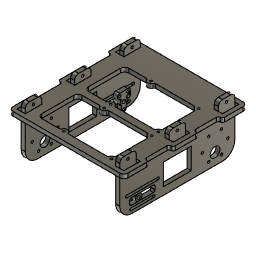
scocca v1.4 (Autodesk Fusion 360 design; units mm, degrees)
Autodesk Fusion 360 part; units mm, degrees
sketch "Schizzo1" plane through (0, 0, 0) normal (0, 0, 1) x (1, 0, 0)
  circle A0 centre (36.25, 84.4234) radius 1.5
  circle A1 centre (28.5, 71) radius 1.5
  circle A2 centre (36.25, 57.5766) radius 1.5
  circle A3 centre (59.5, 71) radius 1.5
  circle A4 centre (51.75, 57.5766) radius 1.5
  circle A5 centre (51.75, 84.4234) radius 1.5
  circle A6 centre (44, 64) radius 6
  line L0 (19.9998, 100) -> (19.9998, 65)
  line L1 (34.9998, 50) -> (145, 50)
  line L2 (160, 100) -> (160, 65)
  arc A7 (19.9998, 65) -> (34.9998, 50) centre (34.9998, 65) ccw
  arc A8 (145, 50) -> (160, 65) centre (145, 65) ccw
  line L3 (146, 59) -> (119, 59)
  line L4 (117, 61) -> (117, 65)
  line L5 (119, 67) -> (146, 67)
  line L6 (148, 65) -> (148, 61)
  arc A9 (117, 61) -> (119, 59) centre (119, 61) ccw
  arc A10 (119, 67) -> (117, 65) centre (119, 65) ccw
  arc A11 (148, 65) -> (146, 67) centre (146, 65) ccw
  arc A12 (146, 59) -> (148, 61) centre (146, 61) ccw
  line L7 (113.5, 72.5) -> (151.5, 72.5)
  line L8 (151.5, 69.5) -> (113.5, 69.5)
  line L9 (112, 71) -> (112, 71)
  line L10 (118.5, 53.5) -> (146.5, 53.5)
  line L11 (148, 55) -> (148, 55)
  line L12 (146.5, 56.5) -> (118.5, 56.5)
  line L13 (117, 55) -> (117, 55)
  arc A13 (112, 71) -> (113.5, 69.5) centre (113.5, 71) ccw
  arc A14 (113.5, 72.5) -> (112, 71) centre (113.5, 71) ccw
  arc A15 (148, 55) -> (146.5, 56.5) centre (146.5, 55) ccw
  arc A16 (146.5, 53.5) -> (148, 55) centre (146.5, 55) ccw
  arc A17 (117, 55) -> (118.5, 53.5) centre (118.5, 55) ccw
  arc A18 (118.5, 56.5) -> (117, 55) centre (118.5, 55) ccw
  line L14 (153, 71) -> (153, 71)
  arc A19 (153, 71) -> (151.5, 72.5) centre (151.5, 71) ccw
  arc A20 (151.5, 69.5) -> (153, 71) centre (151.5, 71) ccw
  circle A21 centre (175, 63) radius 2
  circle A22 centre (175, 55) radius 1.5
  circle A23 centre (170, 71) radius 1.5
  circle A24 centre (180, 71) radius 1.5
  line L15 (170, 68) -> (170, 68)
  line L16 (170, 74) -> (180, 74)
  line L17 (180, 68) -> (180, 68)
  arc A25 (170, 74) -> (170, 68) centre (170, 71) ccw
  arc A26 (180, 68) -> (180, 74) centre (180, 71) ccw
  arc A27 (172, 55) -> (178, 55) centre (175, 55) ccw
  arc A28 (172, 66) -> (170, 68) centre (170, 66) ccw
  arc A29 (180, 68) -> (178, 66) centre (180, 66) ccw
  line L18 (172, 55) -> (172, 59.6834)
  arc A30 (178.3333, 60.7889) -> (178.2, 65.4) centre (175, 63) ccw
  arc A31 (171.8, 65.4) -> (171.6667, 60.7889) centre (175, 63) ccw
  line L19 (178, 55) -> (178, 59.6834)
  arc A32 (172, 59.6834) -> (171.6667, 60.7889) centre (170, 59.6834) ccw
  arc A33 (178.3333, 60.7889) -> (178, 59.6834) centre (180, 59.6834) ccw
  arc A34 (171.8, 65.4) -> (172, 66) centre (171, 66) ccw
  arc A35 (178, 66) -> (178.2, 65.4) centre (179, 66) ccw
  line L20 (39.9998, 100) -> (39.9998, 110)
  line L21 (34.9998, 115) -> (24.9998, 115)
  line L22 (19.9998, 110) -> (19.9998, 100)
  line L23 (79.9999, 100) -> (79.9999, 110)
  line L24 (84.9999, 115) -> (89.9999, 115)
  line L25 (99.9999, 100) -> (99.9999, 110)
  line L26 (94.9999, 115) -> (89.9999, 115)
  line L27 (145, 115) -> (155, 115)
  line L28 (160, 110) -> (160, 100)
  line L29 (140, 100) -> (140, 110)
  line L30 (140, 100) -> (99.9999, 100)
  line L31 (79.9999, 100) -> (39.9998, 100)
  arc A36 (24.9998, 115) -> (19.9998, 110) centre (24.9998, 110) ccw
  arc A37 (39.9998, 110) -> (34.9998, 115) centre (34.9998, 110) ccw
  arc A38 (84.9999, 115) -> (79.9999, 110) centre (84.9999, 110) ccw
  arc A39 (99.9999, 110) -> (94.9999, 115) centre (94.9999, 110) ccw
  arc A40 (145, 115) -> (140, 110) centre (145, 110) ccw
  arc A41 (160, 110) -> (155, 115) centre (155, 110) ccw
  line L32 (29.9998, 115) -> (29.9998, 110)
  circle A42 centre (29.9998, 110) radius 1.5
  circle A43 centre (89.9999, 110) radius 1.5
  circle A44 centre (150, 110) radius 1.5
  circle A45 centre (30, 95) radius 1.5
  circle A46 centre (89.9999, 95) radius 1.5
  circle A47 centre (150, 95) radius 1.5
  arc A48 (10, 280) -> (5, 275) centre (10, 275) ccw
  arc A49 (5, 135) -> (10, 130) centre (10, 135) ccw
  line L33 (10, 135) -> (20, 135)
  line L34 (20, 135) -> (20, 155)
  line L35 (20, 155) -> (10, 155)
  line L36 (10, 155) -> (10, 135)
  line L37 (20, 205) -> (20, 195)
  line L38 (20, 195) -> (10, 195)
  line L39 (10, 195) -> (10, 205)
  line L40 (20, 205) -> (20, 215)
  line L41 (20, 215) -> (10, 215)
  line L42 (10, 215) -> (10, 205)
  line L43 (20, 275) -> (20, 255)
  line L44 (20, 255) -> (10, 255)
  line L45 (10, 275) -> (20, 275)
  line L46 (10, 255) -> (10, 275)
  line L47 (140, 255) -> (140, 275)
  line L48 (140, 275) -> (130, 275)
  line L49 (130, 275) -> (130, 255)
  line L50 (130, 255) -> (140, 255)
  line L51 (130, 205) -> (130, 195)
  line L52 (130, 195) -> (140, 195)
  line L53 (140, 195) -> (140, 205)
  line L54 (130, 135) -> (130, 155)
  line L55 (130, 155) -> (140, 155)
  line L56 (140, 135) -> (130, 135)
  line L57 (140, 155) -> (140, 135)
  line L58 (130, 205) -> (130, 215)
  line L59 (130, 215) -> (140, 215)
  line L60 (140, 215) -> (140, 205)
  line L61 (10, 162.5) -> (10, 187.5)
  line L62 (-2.5, 160) -> (-2.5, 160)
  line L63 (-2.5, 190) -> (-2.5, 190)
  line L64 (-2.5, 220) -> (-2.5, 220)
  line L65 (10, 222.5) -> (10, 247.5)
  line L66 (-2.5, 250) -> (-2.5, 250)
  line L67 (5, 275) -> (5, 252.5)
  line L68 (5, 217.5) -> (5, 192.5)
  line L69 (5, 157.5) -> (5, 135)
  arc A50 (7.5, 160) -> (5, 157.5) centre (7.5, 157.5) ccw
  arc A51 (7.5, 160) -> (10, 162.5) centre (7.5, 162.5) ccw
  arc A52 (10, 187.5) -> (7.5, 190) centre (7.5, 187.5) ccw
  arc A53 (5, 192.5) -> (7.5, 190) centre (7.5, 192.5) ccw
  arc A54 (5, 252.5) -> (7.5, 250) centre (7.5, 252.5) ccw
  arc A55 (10, 247.5) -> (7.5, 250) centre (7.5, 247.5) ccw
  arc A56 (7.5, 220) -> (10, 222.5) centre (7.5, 222.5) ccw
  arc A57 (7.5, 220) -> (5, 217.5) centre (7.5, 217.5) ccw
  arc A58 (145, 275) -> (140, 280) centre (140, 275) ccw
  line L70 (145, 275) -> (145, 252.5)
  arc A59 (142.5, 250) -> (145, 252.5) centre (142.5, 252.5) ccw
  line L71 (152.5, 250) -> (152.5, 250)
  arc A60 (142.5, 250) -> (140, 247.5) centre (142.5, 247.5) ccw
  line L72 (140, 222.5) -> (140, 247.5)
  arc A61 (140, 222.5) -> (142.5, 220) centre (142.5, 222.5) ccw
  line L73 (152.5, 220) -> (152.5, 220)
  arc A62 (145, 217.5) -> (142.5, 220) centre (142.5, 217.5) ccw
  line L74 (145, 217.5) -> (145, 192.5)
  arc A63 (142.5, 190) -> (145, 192.5) centre (142.5, 192.5) ccw
  line L75 (152.5, 190) -> (152.5, 190)
  arc A64 (142.5, 190) -> (140, 187.5) centre (142.5, 187.5) ccw
  line L76 (140, 162.5) -> (140, 187.5)
  arc A65 (140, 162.5) -> (142.5, 160) centre (142.5, 162.5) ccw
  line L77 (152.5, 160) -> (152.5, 160)
  arc A66 (145, 157.5) -> (142.5, 160) centre (142.5, 157.5) ccw
  line L78 (145, 157.5) -> (145, 135)
  arc A67 (140, 130) -> (145, 135) centre (140, 135) ccw
  line L79 (10, 280) -> (140, 280)
  line L80 (10, 130) -> (140, 130)
  circle A68 centre (62, 189) radius 1.25
  circle A69 centre (62, 140) radius 1.25
  circle A70 centre (120, 189) radius 1.25
  circle A71 centre (120, 140) radius 1.25
  line L81 (30, 145) -> (30, 184)
  line L82 (120, 183.3431) -> (120, 145.6569)
  arc A72 (58.2288, 187.6667) -> (65.7712, 187.6667) centre (62, 189) ccw
  line L83 (35, 189) -> (56.3431, 189)
  line L84 (56.3431, 140) -> (35, 140)
  arc A73 (65.7712, 141.3333) -> (58.2288, 141.3333) centre (62, 140) ccw
  arc A74 (118.6667, 143.7712) -> (116.2288, 141.3333) centre (120, 140) ccw
  line L85 (114.3431, 140) -> (67.6569, 140)
  arc A75 (116.2288, 187.6667) -> (118.6667, 185.2288) centre (120, 189) ccw
  line L86 (67.6569, 189) -> (114.3431, 189)
  arc A76 (58.2288, 187.6667) -> (56.3431, 189) centre (56.3431, 187) ccw
  arc A77 (67.6569, 189) -> (65.7712, 187.6667) centre (67.6569, 187) ccw
  arc A78 (56.3431, 140) -> (58.2288, 141.3333) centre (56.3431, 142) ccw
  arc A79 (65.7712, 141.3333) -> (67.6569, 140) centre (67.6569, 142) ccw
  arc A80 (114.3431, 140) -> (116.2288, 141.3333) centre (114.3431, 142) ccw
  arc A81 (118.6667, 143.7712) -> (120, 145.6569) centre (118, 145.6569) ccw
  arc A82 (120, 183.3431) -> (118.6667, 185.2288) centre (118, 183.3431) ccw
  arc A83 (116.2288, 187.6667) -> (114.3431, 189) centre (114.3431, 187) ccw
  arc A84 (35, 189) -> (30, 184) centre (35, 184) ccw
  arc A85 (30, 145) -> (35, 140) centre (35, 145) ccw
  arc A86 (116.2288, 244.6667) -> (118.6667, 242.2288) centre (120, 246) ccw
  line L87 (114.3431, 197) -> (67.6569, 197)
  arc A87 (65.7712, 198.3333) -> (67.6569, 197) centre (67.6569, 199) ccw
  line L88 (120, 240.3431) -> (120, 202.6569)
  circle A88 centre (120, 197) radius 1.25
  arc A89 (118.6667, 200.7712) -> (120, 202.6569) centre (118, 202.6569) ccw
  circle A90 centre (62, 197) radius 1.25
  circle A91 centre (62, 246) radius 1.25
  arc A92 (56.3431, 197) -> (58.2288, 198.3333) centre (56.3431, 199) ccw
  line L89 (30, 202) -> (30, 241)
  line L90 (35, 246) -> (56.3431, 246)
  arc A93 (65.7712, 198.3333) -> (58.2288, 198.3333) centre (62, 197) ccw
  arc A94 (114.3431, 197) -> (116.2288, 198.3333) centre (114.3431, 199) ccw
  line L91 (56.3431, 197) -> (35, 197)
  line L92 (67.6569, 246) -> (114.3431, 246)
  arc A95 (58.2288, 244.6667) -> (65.7712, 244.6667) centre (62, 246) ccw
  arc A96 (58.2288, 244.6667) -> (56.3431, 246) centre (56.3431, 244) ccw
  arc A97 (116.2288, 244.6667) -> (114.3431, 246) centre (114.3431, 244) ccw
  arc A98 (35, 246) -> (30, 241) centre (35, 241) ccw
  arc A99 (118.6667, 200.7712) -> (116.2288, 198.3333) centre (120, 197) ccw
  circle A100 centre (120, 246) radius 1.25
  arc A101 (30, 202) -> (35, 197) centre (35, 202) ccw
  arc A102 (120, 240.3431) -> (118.6667, 242.2288) centre (118, 240.3431) ccw
  arc A103 (67.6569, 246) -> (65.7712, 244.6667) centre (67.6569, 244) ccw
  line L93 (72.9999, 85) -> (106.9999, 85)
  line L94 (106.9999, 85) -> (106.9999, 59)
  line L95 (106.9999, 59) -> (72.9999, 59)
  line L96 (72.9999, 59) -> (72.9999, 85)
  dimension "d27" = 3
  dimension "d28" = 3
  dimension "d29" = 12
  dimension "d32" = 15
  dimension "d38" = 1.5
  dimension "d40" = 1.5
  dimension "d41" = 1.5
  dimension "d43" = 4
  dimension "d44" = 3
  dimension "d52" = 2
  dimension "d53" = 2
  dimension "d67" = 2
  dimension "d68" = 1
  dimension "d73" = 5
  dimension "d74" = 3
  dimension "d75" = 3
  dimension "d76" = 3
  dimension "d77" = 3
  dimension "d115" = 2.5
  dimension "d116" = 2.5
  dimension "d117" = 2.5
  dimension "d118" = 2.5
  dimension "d119" = 2.5
  dimension "d120" = 2.5
  dimension "d121" = 2.5
  dimension "d129" = 2.5
  dimension "d135" = 2
  dimension "d136" = 5
  dimension "d137" = 2.5
  dimension "d138" = 2
  dimension "d139" = 5
  dimension "d141" = 34
  dimension "d142" = 26
  constraint perpendicular L0 L30
  constraint perpendicular L0 L1
  constraint tangent L0 A7
  constraint tangent L1 A7
  constraint tangent L1 A8
  constraint tangent L2 A8
  constraint equal A7 A8
  constraint horizontal L3
  constraint vertical L4
  constraint horizontal L5
  constraint tangent L3 A9
  constraint tangent L4 A9
  constraint tangent L4 A10
  constraint tangent L5 A10
  constraint equal A9 A10
  constraint tangent L5 A11
  constraint equal A9 A11
  constraint horizontal L7
  constraint horizontal L8
  constraint horizontal L10
  constraint horizontal L12
  constraint tangent L8 A13
  constraint tangent L7 A14
  constraint equal A13 A14
  constraint tangent L12 A15
  constraint tangent L10 A16
  constraint equal A15 A16
  constraint tangent L10 A17
  constraint equal A15 A17
  constraint tangent L12 A18
  constraint equal A15 A18
  constraint tangent L7 A19
  constraint tangent L8 A20
  constraint equal A19 A20
  constraint concentric A23 A25
  constraint tangent A27 L18
  constraint vertical L18
  constraint tangent L16 A26
  constraint tangent A27 L19
  constraint vertical L19
  constraint tangent A28 L18
  constraint tangent A29 L19
  constraint concentric A21 A30
  constraint concentric A30 A31
  constraint tangent L18 A32
  constraint tangent A31 A32
  constraint tangent A30 A33
  constraint tangent L19 A33
  constraint equal A32 A33
  constraint tangent A28 A34
  constraint tangent A31 A34
  constraint tangent A29 A35
  constraint tangent A30 A35
  constraint equal A34 A35
  constraint vertical L20
  constraint horizontal L21
  constraint vertical L22
  constraint vertical L23
  constraint horizontal L24
  constraint collinear L30 L31
  constraint tangent L21 A36
  constraint tangent L22 A36
  constraint tangent L20 A37
  constraint tangent L21 A37
  constraint equal A36 A37
  constraint tangent L24 A38
  constraint tangent L23 A38
  constraint equal A36 A38
  constraint tangent L25 A39
  constraint tangent L26 A39
  constraint equal A36 A39
  constraint tangent L27 A40
  constraint tangent L29 A40
  constraint equal A36 A40
  constraint tangent L27 A41
  constraint tangent L28 A41
  constraint equal A36 A41
  constraint midpoint L21 L32.start
  constraint perpendicular L21 L32
  constraint coincident L32.end A42.centre
  constraint vertical L67
  constraint tangent A48 L67
  constraint tangent A49 L67
  constraint vertical L36
  constraint parallel L61 L67
  constraint collinear L67 L68
  constraint collinear L68 L69
  constraint tangent L69 A50
  constraint tangent L61 A51
  constraint equal A50 A51
  constraint tangent L61 A52
  constraint tangent L68 A53
  constraint tangent L67 A54
  constraint tangent L65 A55
  constraint tangent L65 A56
  constraint tangent L68 A57
  constraint tangent A58 L79
  constraint tangent A67 L80
  constraint vertical L81
  constraint horizontal L83
  constraint vertical L82
  constraint concentric A68 A72
  constraint concentric A70 A75
  constraint concentric A69 A73
  constraint concentric A71 A74
  constraint collinear L83 L86
  constraint tangent A72 A76
  constraint tangent L83 A76
  constraint tangent A72 A77
  constraint tangent L86 A77
  constraint equal A76 A77
  constraint tangent L84 A78
  constraint tangent A73 A78
  constraint equal A76 A78
  constraint tangent A73 A79
  constraint tangent L85 A79
  constraint equal A76 A79
  constraint tangent A74 A80
  constraint tangent L85 A80
  constraint equal A76 A80
  constraint tangent A74 A81
  constraint tangent L82 A81
  constraint equal A76 A81
  constraint tangent A75 A82
  constraint tangent L82 A82
  constraint equal A76 A82
  constraint tangent A75 A83
  constraint tangent L86 A83
  constraint equal A76 A83
  constraint tangent L81 A84
  constraint tangent L83 A84
  constraint tangent L81 A85
  constraint tangent L84 A85
  constraint equal A84 A85
  constraint vertical L89
  constraint horizontal L90
  constraint vertical L88
  constraint concentric A91 A95
  constraint concentric A86 A100
  constraint concentric A90 A93
  constraint concentric A88 A99
  constraint collinear L90 L92
  constraint tangent A95 A96
  constraint tangent L90 A96
  constraint tangent A95 A103
  constraint tangent L92 A103
  constraint equal A96 A103
  constraint tangent A92 L91
  constraint tangent A92 A93
  constraint equal A92 A96
  constraint tangent A87 A93
  constraint tangent L87 A87
  constraint equal A87 A96
  constraint tangent A94 A99
  constraint tangent L87 A94
  constraint equal A94 A96
  constraint tangent A89 A99
  constraint tangent L88 A89
  constraint equal A89 A96
  constraint tangent A86 A102
  constraint tangent L88 A102
  constraint equal A96 A102
  constraint tangent A86 A97
  constraint tangent L92 A97
  constraint equal A96 A97
  constraint tangent L89 A98
  constraint tangent L90 A98
  constraint tangent L89 A101
  constraint tangent L91 A101
  constraint equal A98 A101
  constraint horizontal L93
  constraint vertical L94
  constraint horizontal L95
  constraint vertical L96
  measures "d27" diameter of A0
  measures "d28" diameter of A1
  measures "d29" diameter of A6
  measures "d32" radius of A7
  measures "d38" radius of A13
  measures "d40" radius of A15
  measures "d41" radius of A19
  measures "d43" diameter of A21
  measures "d44" diameter of A22
  measures "d52" radius of A28
  measures "d53" radius of A29
  measures "d67" radius of A32
  measures "d68" radius of A34
  measures "d73" radius of A36
  measures "d74" diameter of A42
  measures "d75" diameter of A43
  measures "d76" diameter of A44
  measures "d77" diameter of A45
  measures "d115" radius of A50
  measures "d116" radius of A52
  measures "d117" radius of A53
  measures "d118" radius of A54
  measures "d119" radius of A55
  measures "d120" radius of A56
  measures "d121" radius of A57
  measures "d129" diameter of A71
  measures "d135" radius of A76
  measures "d136" radius of A84
  measures "d137" diameter of A88
  measures "d138" radius of A96
  measures "d139" radius of A98
  measures "d141" distance of L93.start L93.end
  measures "d142" distance of L93.start L95.end
extrude "Extrude1" add sketch "Schizzo1" along normal blind 5 makes body 1 at (70.7954, 265.7296, 0) makes body 2 at (137.954, 79.6743, 0) makes body 3 at (173.8942, 69.399, 0)
sketch "Sketch2" plane through (0, 0, 5) normal (0, 0, 1) x (-1, 0, 0)
  circle A0 centre (-170, -71) radius 1.5
  circle A1 centre (-180, -71) radius 1.5
  circle A2 centre (-175, -55) radius 1.5
  circle A3 centre (-175, -63) radius 2
  arc A4 (-180, -68) -> (-180, -74) centre (-180, -71) ccw
  line L0 (-180, -74) -> (-170, -74)
  arc A5 (-170, -74) -> (-170, -68) centre (-170, -71) ccw
  arc A6 (-172, -66) -> (-170, -68) centre (-170, -66) ccw
  arc A7 (-171.8, -65.4) -> (-172, -66) centre (-171, -66) ccw
  arc A8 (-171.8, -65.4) -> (-171.6667, -60.7889) centre (-175, -63) ccw
  arc A9 (-172, -59.6834) -> (-171.6667, -60.7889) centre (-170, -59.6834) ccw
  line L1 (-172, -59.6834) -> (-172, -55)
  arc A10 (-172, -55) -> (-178, -55) centre (-175, -55) ccw
  line L2 (-178, -55) -> (-178, -59.6834)
  arc A11 (-178.3333, -60.7889) -> (-178, -59.6834) centre (-180, -59.6834) ccw
  arc A12 (-178.3333, -60.7889) -> (-178.2, -65.4) centre (-175, -63) ccw
  arc A13 (-178, -66) -> (-178.2, -65.4) centre (-179, -66) ccw
  arc A14 (-180, -68) -> (-178, -66) centre (-180, -66) ccw
  circle A15 centre (-175, -63) radius 2
  circle A16 centre (-175, -63) radius 4
  constraint concentric A3 A15
  constraint concentric A15 A16
extrude "Extrude2" add sketch "Sketch2" along normal blind 5 contours A8 A12 A16 bodies 3
move_body "Move1" bodies 2 to x (0, 1, 0) y (0, 0, 1) z (1, 0, 0) at (4.9998, 115.0002, -100)
copy_body "CopyPasteBodies1" bodies 2 makes body 4
move_body "Move2" bodies 4 to x (1, 0, 0) y (0, 1, 0) z (0, 0, 1) at (135, 0, 0)
move_body "Move3" bodies 4 to x (-1, 0, 0) y (0, -1, 0) z (0, 0, 1) at (279.9995, 270, 0)
move_body "Move4" bodies 4 to x (1, 0, 0) y (0, 1, 0) z (0, 0, 1) at (-2.4998, 140.0001, 0)
move_body "Move5" bodies 3 to x (0, -1, 0) y (0, 0, 1) z (-1, 0, 0) at (167, 219, -52)
move_body "Move6" bodies 3 to x (1, 0, 0) y (0, 1, 0) z (0, 0, 1) at (-152, 206, -48)
copy_body "CopyPasteBodies2" bodies 3 makes body 5
move_body "Move7" bodies 5 to x (-1, 0, 0) y (0, -1, 0) z (0, 0, 1) at (150, 408, 0)
move_body "Move8" bodies 4 to x (1, 0, 0) y (0, 1, 0) z (0, 0, 1) at (-2.5, 0, 0)
move_body "Move9" bodies 2 to x (1, 0, 0) y (0, 1, 0) z (0, 0, 1) at (5, 0, 0)
move_body "Move10" bodies 2 to x (1, 0, 0) y (0, 1, 0) z (0, 0, 1) at (5, 0, 0)
move_body "Move11" bodies 5 to x (1, 0, 0) y (0, 1, 0) z (0, 0, 1) at (-10, 0, 0)
move_body "Move12" bodies 3 to x (1, 0, 0) y (0, 1, 0) z (0, 0, 1) at (10, 0, 0)
